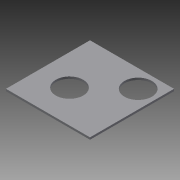
# Autodesk Inventor part: Element
Saved by Autodesk Inventor 2015 (Build 190159000, 159)
## iProperties
Created: 2016-03-23
Part Number: Element
Material: Generic
Document SubType Name: Modeling
Designer: Noah
Density: 1 g/cm^3
Appearance: Default
Author: Noah
Autodesk Inventor part; units mm, degrees
ref_plane "YZ Plane" through (0, 0, 0) normal (1, 0, 0) x (0, 1, 0)
ref_plane "XZ Plane" through (0, 0, 0) normal (0, 1, 0) x (-1, 0, 0)
ref_plane "XY Plane" through (0, 0, 0) normal (0, 0, 1) x (1, 0, 0)
sketch "Sketch1" plane through (0, 0, 0) normal (0, 0, 1) x (1, 0, 0)
  line L0 (-172, 172) -> (172, 172)
  line L1 (172, 172) -> (172, -172)
  line L2 (172, -172) -> (-172, -172)
  line L3 (-172, -172) -> (-172, 172)
  point P0 (0, 0)
  dimension "d0" = 344
  dimension "d1" = 344
  dimension "d2" = 172
  dimension "d3" = 172
  constraints: 8 end point, 2 parallel, 1 horizontal, 1 perpendicular
  measures "d0" distance of L0.start L0.end
  measures "d1" distance of L2.end L0.start
  measures "d2" distance from line of point (0, 0) L1
  measures "d3" distance from line of point (0, 0) L0
extrude "Extrusion1" add sketch "Sketch1" along normal blind 8
sketch "Sketch3" plane through (0, 0, 0) normal (0, 0, -1) x (-1, 0, 0)
  circle A0 centre (-102, 102) radius 53.5
  circle A1 centre (52, -28) radius 53.5
  circle A2 centre (52, -28) radius 12.5 construction
  circle A3 centre (-102, 102) radius 12.5 construction
  point P0 (0, 0)
  dimension "d18" = 107
  dimension "d19" = 107
  constraints: 2 centre point, 2 concentric
  measures "d18" diameter of A1
  measures "d19" diameter of A0
extrude "Extrusion2" cut sketch "Sketch3" against normal through all
sketch "Sketch4" plane through (0, 0, 0) normal (0, 0, -1) x (-1, 0, 0)
  line L0 (118.61, 61.21) -> (118.61, -90.79) projected
  line L1 (119.61, -91.79) -> (167.35, -91.79) projected
  line L2 (168.35, -90.79) -> (168.35, 61.21) projected
  line L3 (167.35, 62.21) -> (119.61, 62.21) projected
  line L4 (162, 69.21) -> (63.35, 69.21) projected
  line L5 (63.35, 106.21) -> (162, 106.21) projected
  line L6 (63.35, 69.21) -> (63.35, 106.21) projected
  line L7 (163.35, 69.21) -> (163.35, 106.21) projected
  arc A0 (118.61, -90.79) -> (119.61, -91.79) centre (119.61, -90.79) ccw projected
  arc A1 (167.35, -91.79) -> (168.35, -90.79) centre (167.35, -90.79) ccw projected
  arc A2 (168.35, 61.21) -> (167.35, 62.21) centre (167.35, 61.21) ccw projected
  arc A3 (119.61, 62.21) -> (118.61, 61.21) centre (119.61, 61.21) ccw projected
  line L8 (162, 69.21) -> (163.35, 69.21) projected
  line L9 (163.35, 106.21) -> (162, 106.21) projected
  point P0 (0, 0)
extrude "Extrusion3" cut sketch "Sketch4" against normal through all
sketch "Sketch5" plane through (0, 0, 0) normal (0, 0, -1) x (-1, 0, 0)
  line L0 (-87, -15) -> (-87, -163) construction
  line L1 (-171, -15) -> (-87, -15) construction
  line L2 (-171, -163) -> (-171, -15) construction
  line L3 (-87, -163) -> (-171, -163) construction
  line L4 (-91, -154) -> (-91, -24)
  line L5 (-96, -19) -> (-162, -19)
  line L6 (-167, -24) -> (-167, -154)
  line L7 (-162, -159) -> (-96, -159)
  arc A0 (-96, -159) -> (-91, -154) centre (-96, -154) ccw
  arc A1 (-167, -154) -> (-162, -159) centre (-162, -154) ccw
  arc A2 (-162, -19) -> (-167, -24) centre (-162, -24) ccw
  arc A3 (-91, -24) -> (-96, -19) centre (-96, -24) ccw
  point P0 (0, 0)
  dimension "d20" = 4
  dimension "d21" = 5
  constraints: 8 end point, 8 point on circle, 8 tangent, 4 centre point, 3 equal radius, 3 other
  measures "d20" distance between parallel lines of L0 L4
  measures "d21" radius of A0
extrude "Extrusion4" cut sketch "Sketch5" against normal through all
equation "\"d0\" = edge_length - 2 * wall_width"
equation "\"d1\" = edge_length - 2 * wall_width"
equation "\"d2\" = -wall_width + 0.5 * edge_length"
equation "\"d3\" = -wall_width + 0.5 * edge_length"
equation "\"d4\" = wall_width_small"
equation "\"edge_length\" = 360"
equation "\"wall_width\" = 8"
equation "\"wall_width_small\" = 8"
body "Solid1"
